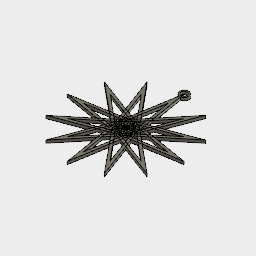
挂件 v1 (Autodesk Fusion 360 design; units mm, degrees)
Autodesk Fusion 360 part; units mm, degrees
sketch "草图1" plane through (0, 0, 0) normal (0, 1, 0) x (1, 0, 0)
  line L0 (-10, 0) -> (0, 60)
  line L1 (0, 60) -> (10, 0)
  line L2 (-5, 2) -> (7, 2)
  line L3 (7, 2) -> (0.1248, 43.2509)
  line L4 (0.1248, 43.2509) -> (-7, 2)
  line L5 (-7, 2) -> (-5, 2)
  line L6 (10, 0) -> (-10, 0)
extrude "拉伸1" add sketch "草图1" along normal blind 3 makes body 1
pattern_circular "C-阵列1" count 12 over 360 about axis through (0, 1.75, 0) along (0, 1, 0) of bodies 1 makes body 2 at (-20.0592, 0, -28.1601) makes body 3 at (-31.4518, 0, -14.3578) makes body 4 at (-34.417, 0, 3.2917) makes body 5 at (-28.1601, 0, 20.0592) makes body 6 at (-14.3578, 0, 31.4518) makes body 7 at (3.2917, 0, 34.417) makes body 8 at (20.0592, 0, 28.1601) makes body 9 at (31.4518, 0, 14.3578) makes body 10 at (34.417, 0, -3.2917) makes body 11 at (28.1601, 0, -20.0592) makes body 12 at (14.3578, 0, -31.4518)
sketch "草图2" plane through (0, 3, 0) normal (0, 1, 0) x (-1, 0, 0)
  line L0 (-7, -2) -> (7, -2)
  line L1 (7, -2) -> (-0.1248, -43.2509)
  line L2 (-0.1248, -43.2509) -> (-7, -2)
  line L3 (-10, 0) -> (0, -60)
  line L4 (0, -60) -> (10, 0)
  line L5 (10, 0) -> (-10, 0)
  circle A0 centre (0, -60) radius 4.7063
  circle A1 centre (0, -60) radius 3.1623
extrude "拉伸2" add sketch "草图2" against normal blind 3 contours L3 L4 A0 A1 picked at (4.1634, -60.3834) bodies 1
